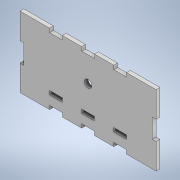
# Autodesk Inventor part: Стенка t2
Saved by Autodesk Inventor 2021 (Build 250183000, 183)
## iProperties
Created: 2021-04-11
Part Number: Стенка t2
Material: Типовые
Document SubType Name: Modeling
Designer: user
Density: 1 g/cm^3
Appearance: По умолчанию
Author: user
Autodesk Inventor part; units mm, degrees
ref_plane "YZ Plane" through (0, 0, 0) normal (1, 0, 0) x (0, 1, 0)
ref_plane "XZ Plane" through (0, 0, 0) normal (0, 1, 0) x (-1, 0, 0)
ref_plane "XY Plane" through (0, 0, 0) normal (0, 0, 1) x (1, 0, 0)
sketch "Эскиз1" plane through (0, 0, 0) normal (0, 0, 1) x (1, 0, 0)
  line L0 (-20, -22.5) -> (-20, -19.5)
  line L1 (-20, -19.5) -> (-30, -19.5)
  line L2 (-30, -19.5) -> (-30, -22.5)
  line L3 (0, -19.5) -> (-5, -19.5)
  line L4 (-5, -19.5) -> (-5, -22.5)
  line L5 (20, -22.5) -> (20, -19.5)
  line L6 (20, -19.5) -> (30, -19.5)
  line L7 (30, -19.5) -> (30, -22.5)
  line L8 (0, -19.5) -> (5, -19.5)
  line L9 (5, -19.5) -> (5, -22.5)
  line L10 (-53, 22.5) -> (-30, 22.5)
  line L11 (-20, 22.5) -> (-20, 19.5)
  line L12 (-20, 19.5) -> (-30, 19.5)
  line L13 (-30, 19.5) -> (-30, 22.5)
  line L14 (-20, 22.5) -> (-5, 22.5)
  line L15 (0, 19.5) -> (-5, 19.5)
  line L16 (-5, 19.5) -> (-5, 22.5)
  line L17 (-5, 22.5) -> (-20, 22.5)
  line L18 (-30, 22.5) -> (-53, 22.5)
  line L19 (53, 22.5) -> (30, 22.5)
  line L20 (20, 22.5) -> (20, 19.5)
  line L21 (20, 19.5) -> (30, 19.5)
  line L22 (30, 19.5) -> (30, 22.5)
  line L23 (20, 22.5) -> (5, 22.5)
  line L24 (0, 19.5) -> (5, 19.5)
  line L25 (5, 19.5) -> (5, 22.5)
  line L26 (5, 22.5) -> (20, 22.5)
  line L27 (30, 22.5) -> (53, 22.5)
  line L28 (-20, -32.5) -> (-20, -29.5)
  line L29 (-20, -29.5) -> (-30, -29.5)
  line L30 (-30, -29.5) -> (-30, -32.5)
  line L31 (5, -32.5) -> (5, -29.5)
  line L32 (5, -29.5) -> (-5, -29.5)
  line L33 (-5, -29.5) -> (-5, -32.5)
  line L34 (30, -32.5) -> (30, -29.5)
  line L35 (30, -29.5) -> (20, -29.5)
  line L36 (20, -29.5) -> (20, -32.5)
  line L37 (-30, -22.5) -> (-20, -22.5)
  line L38 (-5, -22.5) -> (5, -22.5)
  line L39 (20, -22.5) -> (30, -22.5)
  line L40 (-30, -32.5) -> (-53, -32.5)
  line L41 (-5, -32.5) -> (-20, -32.5)
  line L42 (53, -32.5) -> (30, -32.5)
  line L43 (20, -32.5) -> (5, -32.5)
  line L44 (-53, 2.5) -> (-50, 2.5)
  line L45 (-50, 2.5) -> (-50, -12.5)
  line L46 (-50, -12.5) -> (-53, -12.5)
  line L47 (53, 2.5) -> (50, 2.5)
  line L48 (50, 2.5) -> (50, -12.5)
  line L49 (50, -12.5) -> (53, -12.5)
  line L50 (-53, 22.5) -> (-53, 2.5)
  line L51 (-53, -12.5) -> (-53, -32.5)
  line L52 (53, -32.5) -> (53, -12.5)
  line L53 (53, 2.5) -> (53, 22.5)
  circle A0 centre (0, 0) radius 3
  dimension "d15" = 6
  constraints: 108 end point, 12 equal length, 4 perpendicular, 3 horizontal, 1 centre point, 1 coincident
  measures "d15" diameter of A0
extrude "Выдавливание1" add sketch "Эскиз1" along normal blind 3
